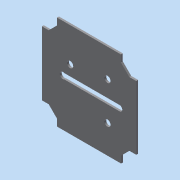
# Autodesk Inventor part: 20_Cube_insert_AlliedVision_Alvium_v3
Saved by Autodesk Inventor 2019.4 (Build 234330000, 330)
## iProperties
Created: 2019-08-07
Part Number: 20_Cube_insert_AlliedVision_Alvium_v3
Material: Generic
Document SubType Name: Modeling
Designer: marsikovabarbora
Density: 1 g/cm^3
Appearance: Default
Author: marsikovabarbora
Autodesk Inventor part; units mm, degrees
ref_plane "YZ Plane" through (0, 0, 0) normal (1, 0, 0) x (0, 1, 0)
ref_plane "XZ Plane" through (0, 0, 0) normal (0, 1, 0) x (-1, 0, 0)
ref_plane "XY Plane" through (0, 0, 0) normal (0, 0, 1) x (1, 0, 0)
ref_plane "Work Plane1" through (-29.1, -14.5, 2.4) normal (0, 0, -1) x (0, 1, 0)
ref_plane "Work Plane2" through (-13.8999, -10.5497, 2.25) normal (0, 0, -1) x (0, 1, 0)
sketch "Sketch1" plane through (0, 0, 0) normal (0, 0, 1) x (1, 0, 0)
  line L0 (-34.86, 0) -> (34.86, 0) construction
  line L1 (0, -34.86) -> (0, 34.86) construction
  line L2 (0, 0) -> (11.1575, 11.1575) construction
  line L3 (0, 0) -> (15.7791, 0) construction
  line L4 (0, 24.9) -> (16.8009, 24.9)
  line L5 (16.8009, 24.9) -> (16.8009, 21.2415)
  line L6 (16.8009, 21.2415) -> (19.0212, 19.0212)
  line L7 (24.9, 0) -> (24.9, 16.8009)
  line L8 (24.9, 16.8009) -> (21.2415, 16.8009)
  line L9 (21.2415, 16.8009) -> (19.0212, 19.0212)
  line L10 (0, -24.9) -> (16.8009, -24.9)
  line L11 (16.8009, -24.9) -> (16.8009, -21.2415)
  line L12 (16.8009, -21.2415) -> (19.0212, -19.0212)
  line L13 (24.9, 0) -> (24.9, -16.8009)
  line L14 (24.9, -16.8009) -> (21.2415, -16.8009)
  line L15 (21.2415, -16.8009) -> (19.0212, -19.0212)
  line L16 (0, 24.9) -> (-16.8009, 24.9)
  line L17 (-16.8009, 24.9) -> (-16.8009, 21.2415)
  line L18 (-16.8009, 21.2415) -> (-19.0212, 19.0212)
  line L19 (-24.9, 16.8009) -> (-21.2415, 16.8009)
  line L20 (-21.2415, 16.8009) -> (-19.0212, 19.0212)
  line L21 (0, -24.9) -> (-16.8009, -24.9)
  line L22 (-16.8009, -24.9) -> (-16.8009, -21.2415)
  line L23 (-16.8009, -21.2415) -> (-19.0212, -19.0212)
  line L24 (-21.2415, -16.8009) -> (-19.0212, -19.0212)
  line L25 (-24.9, -16.8009) -> (-21.2415, -16.8009)
  line L26 (-24.9, 0) -> (-24.9, -16.8009)
  line L27 (-24.9, 0) -> (-24.9, 16.8009)
  circle A0 centre (0, 0) radius 10
  dimension "d0" = 45
  dimension "d2" = 24.9
  dimension "d3" = 3.14
  dimension "d4" = 26.9
  dimension "d5" = 20
  constraints: 52 end point, 20 symmetric about line, 2 horizontal, 2 perpendicular, 2 point on line, 1 centre point, 1 coincident, 1 equal length
  measures "d0" angle of L3 L2
  measures "d2" distance between parallel lines of L0 L4
  measures "d3" distance of L5.end L6.end
  measures "d4" distance from line of L2.start L6
  measures "d5" diameter of A0
extrude "Extrusion1" add sketch "Sketch1" along normal blind 1 contours L4 L5 L6 L9 L8 L7 L13 L14 L15 L12 L11 L10 L21 L22 L23 L24 L25 L26 L27 L19 L20 L18 L17 L16 | A0
sketch "Sketch5" plane through (0, 0, 0) normal (0, 0, -1) x (-1, 0, 0)
  circle A0 centre (-9.7, 10) radius 1.4
  circle A1 centre (-9.7, -10) radius 1.4
  circle A2 centre (13.8, 0) radius 1.4
  circle A3 centre (-10, 6.9) radius 0.75
  circle A4 centre (10, 6.9) radius 1.25
  point P0 (0, 0)
  constraints: 5 centre point, 10 other
hole "Hole1" at (-13.8, 0, 0) at (9.7, -10, 0) at (-10, 6.9, 0) at (9.7, 10, 0) direction (0, 0, 1) diameter 3.3 depth 12 tip angle 118
sketch "Skizze6" plane through (-16.8009, 24.9, 1) normal (0, 0, 1) x (1, 0, 0)
  circle A0 centre (6.8009, -18) radius 1.65 construction
  circle A1 centre (3.0009, -24.9) radius 1.65 construction
  circle A2 centre (26.5009, -34.9) radius 1.65 construction
  circle A3 centre (26.5009, -14.9) radius 1.65 construction
  line L0 (33.6017, -3.6585) -> (33.6017, 0) projected
  line L1 (33.6017, 0) -> (0, 0) construction
  line L2 (0, 0) -> (0, -3.6585) projected
  line L3 (0, -3.6585) -> (-4.4406, -8.0991) projected
  line L4 (-4.4406, -8.0991) -> (-8.0991, -8.0991) projected
  line L5 (-8.0991, -8.0991) -> (-8.0991, -41.7009) construction
  line L6 (-8.0991, -41.7009) -> (-4.4406, -41.7009) projected
  line L7 (-4.4406, -41.7009) -> (0, -46.1415) projected
  line L8 (0, -46.1415) -> (0, -49.8) projected
  line L9 (0, -49.8) -> (33.6017, -49.8) construction
  line L10 (33.6017, -49.8) -> (33.6017, -46.1415) projected
  line L11 (33.6017, -46.1415) -> (38.0423, -41.7009) projected
  line L12 (38.0423, -41.7009) -> (41.7009, -41.7009) projected
  line L13 (41.7009, -41.7009) -> (41.7009, -8.0991) construction
  line L14 (41.7009, -8.0991) -> (38.0423, -8.0991) projected
  line L15 (38.0423, -8.0991) -> (33.6017, -3.6585) projected
  line L16 (-0.1, 0.1) -> (33.7017, 0.1) construction
  line L17 (33.7017, 0.1) -> (33.7017, -3.6171)
  line L18 (33.7017, -3.6171) -> (38.0838, -7.9991)
  line L19 (38.0838, -7.9991) -> (41.8009, -7.9991)
  line L20 (41.8009, -7.9991) -> (41.8009, -41.8009) construction
  line L21 (41.8009, -41.8009) -> (38.0838, -41.8009)
  line L22 (38.0838, -41.8009) -> (33.7017, -46.1829)
  line L23 (33.7017, -46.1829) -> (33.7017, -49.9)
  line L24 (33.7017, -49.9) -> (-0.1, -49.9) construction
  line L25 (-0.1, -49.9) -> (-0.1, -46.1829)
  line L26 (-0.1, -46.1829) -> (-4.4821, -41.8009)
  line L27 (-4.4821, -41.8009) -> (-8.1991, -41.8009)
  line L28 (-8.1991, -41.8009) -> (-8.1991, -7.9991) construction
  line L29 (-8.1991, -7.9991) -> (-4.4821, -7.9991)
  line L30 (-4.4821, -7.9991) -> (-0.1, -3.6171)
  line L31 (-0.1, -3.6171) -> (-0.1, 0.1)
  line L32 (-8.0991, -8.0991) -> (-8.0991, -7.9991)
  line L33 (0, 0) -> (-0.1, 0)
  line L34 (33.6017, 0) -> (33.7017, 0)
  line L35 (41.7009, -8.0991) -> (38.0423, -8.0991) projected
  line L36 (41.7009, -8.0991) -> (41.7009, -7.9991)
  line L37 (41.7009, -41.7009) -> (41.7009, -41.8009)
  line L38 (33.6017, -49.8) -> (33.7017, -49.8)
  line L39 (-8.0991, -41.7009) -> (-8.0991, -41.8009)
  line L40 (0, -49.8) -> (-0.1, -49.8)
  point P0 (16.8009, -24.9)
  dimension "d25" = 0.1
  constraints: 48 end point, 12 point on line, 4 perpendicular, 15 other
  measures "d25" distance between parallel lines of L1 L16
extrude "IM_offset" add sketch "Skizze6" against normal blind 1 contours L2 L3 L4 L32 L29 L30 L31 L33 | L6 L7 L8 L40 L25 L26 L27 L39 | L10 L11 L12 L37 L21 L22 L23 L38
sketch "Sketch7" plane through (-24.9, 16.9009, 1) normal (0, 0, 1) x (1, 0, 0)
  circle A0 centre (11.1, -16.9009) radius 1.65 projected
  line L0 (11.1, -16.9009) -> (40.9762, -16.9009) construction
  line L1 (11.1, -18.3509) -> (40.9762, -18.3509)
  line L2 (40.9762, -15.4509) -> (11.1, -15.4509)
  arc A1 (11.1, -15.4509) -> (11.1, -18.3509) centre (11.1, -16.9009) ccw
  arc A2 (40.9762, -18.3509) -> (40.9762, -15.4509) centre (40.9762, -16.9009) ccw
  point P0 (24.9, -16.9009)
  point P1 (26.0381, -16.9009)
  dimension "d28" = 2.9
  constraints: 8 end point, 4 point on circle, 4 tangent, 2 centre point, 1 horizontal, 1 midpoint, 1 parallel
  measures "d28" diameter of A2
extrude "Extrusion6" cut sketch "Sketch7" against normal blind 10 contours A0 L1 A1 L2 | A0 L2 A2 L1 picked at (11.65, -16.9009)
body "Solid1"
